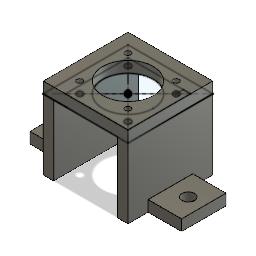
GetShuttleFesting v2 (Autodesk Fusion 360 design; units mm, degrees)
Autodesk Fusion 360 part; units mm, degrees
note: some values were not read from the file. Set by a fixed rule: which sketch regions a step uses.
sketch "Sketch1" plane through (0, 0, 0) normal (0, 1, 0) x (1, 0, 0)
  line L0 (14, 14) -> (-14, 14)
  line L1 (-14, 14) -> (-14, -14)
  line L2 (-14, -14) -> (14, -14)
  line L3 (14, -14) -> (14, 14)
  line L4 (14, 14) -> (-14, -14) construction
  line L5 (-14, 14) -> (14, -14) construction
  line L6 (14, 14) -> (10.8, 14)
  line L7 (10.8, 14) -> (10.8, 10.8)
  circle A0 centre (10.8, 10.8) radius 1.3
  circle A1 centre (-10.8, 10.8) radius 1.3
  circle A2 centre (-10.8, -10.8) radius 1.3
  circle A3 centre (10.8, -10.8) radius 1.3
  line L8 (-19, 19) -> (19, 19)
  line L9 (19, 19) -> (19, -19)
  line L10 (19, -19) -> (-19, -19)
  line L11 (-19, -19) -> (-19, 19)
  line L12 (-19, 19) -> (19, -19) construction
  line L13 (19, 19) -> (-19, -19) construction
  circle A4 centre (0, 0) radius 11.3
  dimension "d1" = 28
  dimension "d2" = 28
  dimension "d3" = 3.2
  dimension "d4" = 3.2
  dimension "d5" = 2.6
  dimension "d7" = 360
  dimension "d8" = 38
  dimension "d9" = 38
  dimension "d10" = 22.6
  constraint horizontal L0
  constraint perpendicular L0 L1
  constraint parallel L0 L2
  constraint parallel L1 L3
  constraint coincident L4 A4.centre
  constraint coincident L5 A4.centre
  constraint coincident A4.centre origin
  constraint coincident L0 L6.end
  constraint perpendicular L0 L7
  constraint coincident L7.end A0.centre
  constraint horizontal L8
  constraint perpendicular L8 L9
  constraint parallel L8 L10
  constraint parallel L9 L11
  constraint coincident L12 A4.centre
  constraint coincident L13 A4.centre
  measures "d1" distance of L1.end L2.end
  measures "d2" distance of L0.end L1.end
  measures "d3" distance of L0.start L6.end
  measures "d4" distance of L6.end L7.end
  measures "d5" diameter of A0
  measures "d8" distance of L9.end L10.end
  measures "d9" distance of L8.end L9.end
  measures "d10" diameter of A4
extrude "Extrude1" add sketch "Sketch1" along normal blind 5 contours L0 L1 L2 L3 L6 | L8 L9 L10 L11
sketch "Sketch2" plane through (0, 0, 0) normal (0, 1, 0) x (1, 0, 0)
  circle A0 centre (10.8, 10.8) radius 1.3
  circle A1 centre (0, 0) radius 11.3
  circle A2 centre (10.8, -10.8) radius 1.3
  circle A3 centre (-10.8, -10.8) radius 1.3
  circle A4 centre (-10.8, 10.8) radius 1.3
  line L0 (19, -19) -> (-19, -19)
  line L1 (-19, -19) -> (-19, 19)
  line L2 (-19, 19) -> (19, 19)
  line L3 (19, 19) -> (19, -19)
  line L4 (14, 19) -> (14, -19)
  line L5 (-14, 19) -> (-14, -19)
  point P0 (-14, -14)
  point P1 (14, -14)
  point P2 (14, 14)
  point P3 (-14, 14)
  constraint coincident L2 L4.start
  constraint coincident L0 L4.end
  constraint perpendicular L0 L4
  constraint coincident L2 L5.start
  constraint coincident L0 L5.end
  constraint perpendicular L0 L5
extrude "Extrude2" add sketch "Sketch2" against normal blind 31.5 contours L0 L2 L3 L4 | L0 L1 L2 L5
extrude "Extrude3" cut 1 faces at (-14, -10.5, -6.3333) along direction (-1, 0, 0) blind 0.3
extrude "Extrude4" cut 1 faces at (14, -10.5, -6.3333) along direction (1, 0, 0) blind 0.3
sketch "Sketch3" plane through (-19, 0, 0) normal (-1, 0, 0) x (0, 0, 1)
  line L0 (19, -31.5) -> (19, 5)
  line L1 (19, 5) -> (-19, 5)
  line L2 (-19, 5) -> (-19, -31.5)
  line L3 (-19, -31.5) -> (19, -31.5)
  line L4 (0, -31.5) -> (-10, -31.5)
  line L5 (0, -31.5) -> (10, -31.5)
  line L6 (10, -31.5) -> (-10, -31.5)
  line L7 (-10, -31.5) -> (-10, -26.5)
  line L8 (-10, -26.5) -> (10, -26.5)
  line L9 (10, -26.5) -> (10, -31.5)
  dimension "d19" = 10
  dimension "d20" = 20
  dimension "d21" = 5
  constraint midpoint L3 L4.start
  constraint coincident L3 L4.end
  constraint perpendicular L2 L4
  constraint perpendicular L2 L5
  constraint horizontal L6
  constraint vertical L7
  constraint horizontal L8
  constraint vertical L9
  measures "d19" distance of L4.start L5.end
  measures "d20" distance of L5.end L4.end
  measures "d21" distance of L5.end L8.end
extrude "Extrude5" add sketch "Sketch3" along normal blind 15 contours L3 L4 L5 L6 L7 L8 L9
sketch "Sketch4" plane through (0, -26.5, 0) normal (0, 1, 0) x (-1, 0, 0)
  line L0 (19, 10) -> (19, -10)
  line L1 (19, -10) -> (34, -10)
  line L2 (34, -10) -> (34, 10)
  line L3 (34, 10) -> (19, 10)
  line L4 (34, 0) -> (27, 0)
  circle A0 centre (27, 0) radius 2.8
  dimension "d24" = 7
  dimension "d25" = 5.6
  constraint midpoint L2 L4.start
  constraint perpendicular L2 L4
  constraint coincident L4.end A0.centre
  measures "d24" distance of L4.start L4.end
  measures "d25" diameter of A0
sketch "Sketch5" plane through (19, 0, 0) normal (1, 0, 0) x (0, 0, -1)
  line L0 (19, -31.5) -> (19, 5)
  line L1 (19, 5) -> (-19, 5)
  line L2 (-19, 5) -> (-19, -31.5)
  line L3 (-19, -31.5) -> (19, -31.5)
  line L4 (0, -31.5) -> (10, -31.5)
  line L5 (10, -31.5) -> (-10, -31.5)
  line L6 (-10, -31.5) -> (-10, -26.5)
  line L7 (-10, -26.5) -> (10, -26.5)
  line L8 (10, -26.5) -> (10, -31.5)
  dimension "d26" = 10
  dimension "d27" = 20
  dimension "d28" = 5
  constraint midpoint L3 L4.start
  constraint parallel L3 L4
  constraint horizontal L5
  constraint vertical L6
  constraint horizontal L7
  constraint vertical L8
  measures "d26" distance of L4.start L4.end
  measures "d27" distance of L4.end L5.end
  measures "d28" distance of L4.end L7.end
extrude "Extrude6" add sketch "Sketch5" along normal blind 15 contours L3 L4 L5 L6 L7 L8
sketch "Sketch6" plane through (0, -26.5, 0) normal (0, 1, 0) x (-1, 0, 0)
  line L0 (-19, -10) -> (-19, 10)
  line L1 (-19, 10) -> (-34, 10)
  line L2 (-34, 10) -> (-34, -10)
  line L3 (-34, -10) -> (-19, -10)
  line L4 (-34, 0) -> (-27, 0)
  circle A0 centre (-27, 0) radius 2.8
  dimension "d31" = 7
  dimension "d32" = 5.6
  constraint midpoint L2 L4.start
  constraint perpendicular L2 L4
  constraint coincident L4.end A0.centre
  measures "d31" distance of L4.start L4.end
  measures "d32" diameter of A0
extrude "Extrude7" cut sketch "Sketch4" sketch "Sketch6" against normal blind 11 contours A0 of sketch 2 contours A0
